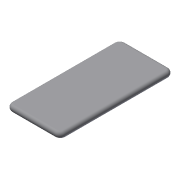
# Autodesk Inventor part: 00_Huawei_P20
Saved by Autodesk Inventor 2019 (Build 230136000, 136)
## iProperties
Created: 2019-08-19
Part Number: 00_Huawei_P20
Material: Generic
Document SubType Name: Modeling
Designer: diederichbenedict
Density: 1 g/cm^3
Appearance: Default
Author: diederichbenedict
Autodesk Inventor part; units mm, degrees
ref_plane "YZ Plane" through (0, 0, 0) normal (1, 0, 0) x (0, 1, 0)
ref_plane "XZ Plane" through (0, 0, 0) normal (0, 1, 0) x (-1, 0, 0)
ref_plane "XY Plane" through (0, 0, 0) normal (0, 0, 1) x (1, 0, 0)
sketch "Sketch1" plane through (0, 0, 0) normal (0, 1, 0) x (-1, 0, 0)
  circle A0 centre (0, 0) radius 4.315
  line L0 (0, 11) -> (0, 22.5) construction
  line L1 (4.315, 11) -> (4.315, 22.5)
  line L2 (-4.315, 22.5) -> (-4.315, 11)
  arc A1 (-4.315, 11) -> (4.315, 11) centre (0, 11) ccw
  arc A2 (4.315, 22.5) -> (-4.315, 22.5) centre (0, 22.5) ccw
  point P0 (0, 16.75)
  dimension "d0" = 8.63
  dimension "d1" = 11.5
  dimension "d2" = 11
  constraints: 8 end point, 4 point on circle, 4 tangent, 3 centre point, 1 coincident, 1 midpoint, 1 parallel, 1 vertical
  measures "d0" diameter of A0
  measures "d1" distance of L0.start L0.end
  measures "d2" distance of point (0, 0) L0.start
extrude "Extrusion1" add sketch "Sketch1" along normal blind 0.5
sketch "Sketch2" plane through (0, 0.5, 0) normal (0, 1, 0) x (1, 0, 0)
  line L0 (-5, -33.5) -> (53.88, -33.5)
  line L1 (61.38, -26) -> (61.38, 114)
  line L2 (53.88, 121.5) -> (-5, 121.5)
  line L3 (-12.5, 114) -> (-12.5, -26)
  circle A0 centre (0, 0) radius 4.315 projected
  line L4 (-4.315, -11) -> (-4.315, -22.5) projected
  arc A1 (4.315, -11) -> (-4.315, -11) centre (0, -11) ccw projected
  line L5 (4.315, -22.5) -> (4.315, -11) projected
  arc A2 (-4.315, -22.5) -> (4.315, -22.5) centre (0, -22.5) ccw projected
  arc A3 (-12.5, -26) -> (-5, -33.5) centre (-5, -26) ccw
  arc A4 (53.88, -33.5) -> (61.38, -26) centre (53.88, -26) ccw
  arc A5 (61.38, 114) -> (53.88, 121.5) centre (53.88, 114) ccw
  arc A6 (-5, 121.5) -> (-12.5, 114) centre (-5, 114) ccw
  point P0 (61.38, 121.5)
  point P1 (-12.5, 121.5)
  dimension "d5" = 73.88
  dimension "d6" = 155
  dimension "d7" = 33.5
  dimension "d8" = 12.5
  dimension "d9" = 7.5
  constraints: 8 end point, 8 point on circle, 8 tangent, 4 centre point, 4 point on line, 3 equal radius, 2 parallel, 1 horizontal, 1 perpendicular
  measures "d5" distance of point (-12.5, 121.5) point (61.38, 121.5)
  measures "d6" distance between parallel lines of L2 L0
  measures "d7" distance from line of L0 point (0, 0)
  measures "d8" distance from line of L3 point (0, 0)
  measures "d9" radius of A3
extrude "Extrusion2" add sketch "Sketch2" along normal blind 8.15 contours A3 L3 A6 L2 A5 L1 A4 L0 | A0 | A1 L5 A2 L4
fillet "Fillet1" radius 4 16 edges at (-10.3033, 0.5, -119.3033) (24.44, 0.5, -121.5) (59.1833, 0.5, -119.3033) (61.38, 0.5, -44) (59.1833, 0.5, 31.3033) (24.44, 0.5, 33.5) (-10.3033, 0.5, 31.3033) (-12.5, 0.5, -44) (-10.3033, 8.65, 31.3033) (24.44, 8.65, 33.5) (59.1833, 8.65, 31.3033) (61.38, 8.65, -44) (59.1833, 8.65, -119.3033) (24.44, 8.65, -121.5) (-10.3033, 8.65, -119.3033) (-12.5, 8.65, -44)
body "Solid1"
